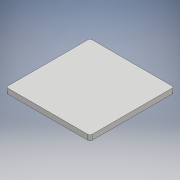
# Autodesk Inventor part: Cap plate
Saved by Autodesk Inventor 2017 (Build 210142000, 142)
## iProperties
Created: 2016-08-05
Part Number: Cap plate
Material: Generic
Document SubType Name: Modeling
Designer: Ali
Density: 1 g/cm^3
Appearance: Default
Author: Ali
## iProperties of the stored document Cap plate_3DPrint.ipt
Created: 2017-01-15
Part Number: Cap plate_3DPrint
Material: Generic
Document SubType Name: Modeling
Designer: Alistair
Density: 1 g/cm^3
Appearance: Default
Author: Alistair
Autodesk Inventor part; units mm, degrees
ref_plane "YZ Plane" through (0, 0, 0) normal (1, 0, 0) x (0, 1, 0)
ref_plane "XZ Plane" through (0, 0, 0) normal (0, 1, 0) x (-1, 0, 0)
ref_plane "XY Plane" through (0, 0, 0) normal (0, 0, 1) x (1, 0, 0)
sketch "Sketch1" plane through (0, 0, 0) normal (0, 0, 1) x (1, 0, 0)
  line L0 (-40, 40) -> (40, 40)
  line L1 (40, 40) -> (40, -40)
  line L2 (40, -40) -> (-40, -40)
  line L3 (-40, -40) -> (-40, 40)
  point P0 (0, 0)
  dimension "d0" = 80
  dimension "d1" = 80
  dimension "d19" = 40
  dimension "d20" = 40
  constraints: 8 end point, 2 parallel, 1 horizontal, 1 perpendicular
  measures "d0" distance of L0.end L1.end
  measures "d1" distance of L1.end L2.end
  measures "d19" distance from line of L3 point (0, 0)
  measures "d20" distance from line of L0 point (0, 0)
extrude "Extrusion1" add sketch "Sketch1" along normal blind 0.3
sketch "Sketch2" plane through (0, 0, 0.3) normal (0, 0, 1) x (1, 0, 0)
  line L0 (40, 40) -> (-40, 40) projected
  line L1 (-40, 40) -> (-40, -40) projected
  line L2 (-40, -40) -> (40, -40) projected
  line L3 (40, -40) -> (40, 40) projected
  line L4 (-41, 41) -> (41, 41)
  line L5 (41, 41) -> (41, -41)
  line L6 (41, -41) -> (-41, -41)
  line L7 (-41, -41) -> (-41, 41)
  point P0 (0, 0)
  dimension "d4" = 1
  constraints: 8 end point, 3 other
  measures "d4" distance between parallel lines of L0 L4
extrude "Extrusion2" add sketch "Sketch2" against normal blind 5
fillet "Fillet1" radius 2 8 edges at (40, 40, -2.35) (-40, 40, -2.35) (40, -40, -2.35) (-40, -40, -2.35) (41, 41, -2.2) (-41, 41, -2.2) (-41, -41, -2.2) (41, -41, -2.2)
sketch "Sketch3" plane through (40, -38, 0) normal (-1, 0, 0) x (0, 0, 1)
  line L0 (-4.7, 77) -> (-4.7, -1) projected
  line L1 (-4.7, 48) -> (-1.7, 48)
  line L2 (-1.7, 48) -> (-1.7, 28)
  line L3 (-1.7, 28) -> (-4.7, 28)
  line L4 (-4.7, 28) -> (-4.7, 48)
  line L5 (0, 78) -> (-4.7, 78) projected
  point P0 (0, 38)
  dimension "d13" = 3
  dimension "d14" = 20
  dimension "d15" = 30
  constraints: 8 end point, 2 parallel, 1 horizontal, 1 perpendicular, 1 point on line
  measures "d13" distance of L2.end L3.end
  measures "d14" distance of L1.end L2.end
  measures "d15" distance between parallel lines of L5 L1
extrude "Extrusion3" add sketch "Sketch3" along normal blind 1.5
chamfer "Chamfer1" distance 1 angle 45 1 edges at (38.5, 0, -1.7)
chamfer "Chamfer2" distance 1 angle 45 1 edges at (38.5, 0, -4.7)
pattern_circular "Circular Pattern1" count 3 over 180 about axis through (0, 0, -10) along (0, 0, 1) of "Extrusion3", "Chamfer2", "Chamfer1"
sketch "Sketch4" plane through (0, 0, -4.7) normal (0, 0, -1) x (-1, 0, 0)
  line L0 (38, -40) -> (-38, -40) projected
  arc A0 (-0.8, -40) -> (0.8, -40) centre (0, -40) ccw
  point P0 (0, 0)
  dimension "d24" = 0.8
  constraints: 2 point on circle, 2 point on line, 1 centre point, 1 midpoint
  measures "d24" radius of A0
extrude "Extrusion4" cut sketch "Sketch4" against normal up to surface (4.7 mm away)
body "Solid1"
